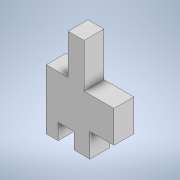
# Autodesk Inventor part: N3
Saved by Autodesk Inventor 2022 (Build 260153000, 153)
## iProperties
Created: 2023-03-30
Part Number: N3
Material: Типовые
Document SubType Name: Modeling
Designer: Arturukis
Density: 1 g/cm^3
Appearance: По умолчанию
Author: Arturukis
Autodesk Inventor part; units mm, degrees
ref_plane "YZ Plane" through (0, 0, 0) normal (1, 0, 0) x (0, 1, 0)
ref_plane "XZ Plane" through (0, 0, 0) normal (0, 1, 0) x (-1, 0, 0)
ref_plane "XY Plane" through (0, 0, 0) normal (0, 0, 1) x (1, 0, 0)
sketch "Эскиз1" plane through (0, 0, 0) normal (0, 0, 1) x (1, 0, 0)
  line L0 (0, 0) -> (6, 0)
  line L1 (6, 0) -> (6, 8)
  line L2 (6, 8) -> (14, 8)
  line L3 (14, 8) -> (14, 0)
  line L4 (14, 0) -> (22, 0)
  line L5 (22, 0) -> (22, 12)
  line L6 (22, 12) -> (34, 12)
  line L7 (34, 12) -> (34, 28)
  line L8 (34, 28) -> (19, 28)
  line L9 (19, 28) -> (19, 50)
  line L10 (19, 50) -> (11, 50)
  line L11 (11, 50) -> (11, 30)
  line L12 (11, 30) -> (0, 30)
  line L13 (0, 30) -> (0, 0)
  line L14 (-6, -4.3803) -> (-6, 17.4799)
  line L15 (-11.9348, 0) -> (0, 0)
  point P0 (-6, 0)
  dimension "d3" = 8
  dimension "d4" = 8
  dimension "d7" = 12
  dimension "d10" = 15
  dimension "d11" = 22
  dimension "d13" = 20
  dimension "d14" = 11
  dimension "d15" = 12
  dimension "d16" = 6
  dimension "d17" = 34
  dimension "d19" = 6
  dimension "d20" = 50
  constraints: 32 end point, 9 perpendicular, 4 horizontal, 2 vertical
  measures "d3" distance of L0.end L1.end
  measures "d4" distance of L1.end L2.end
  measures "d7" distance of L4.end L5.end
  measures "d10" distance of L7.end L8.end
  measures "d11" distance of L8.end L9.end
  measures "d13" distance of L10.end L11.end
  measures "d14" distance of L11.end L12.end
  measures "d15" horizontal distance of L6.end L4.end
  measures "d16" distance from line of L13 L0.end
  measures "d17" horizontal distance of L6.end L0.start
  measures "d19" distance of L0.start point (-6, 0)
  measures "d20" vertical distance of L4.end L9.end
extrude "Выдавливание1" add sketch "Эскиз1" along normal blind 10
